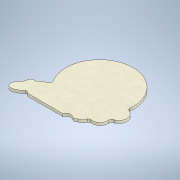
# Autodesk Inventor part: Mirage
Saved by Autodesk Inventor 2021 (Build 250183000, 183)
## iProperties
Created: 2023-03-16
Part Number: Mirage
Material: Paper
Document SubType Name: Modeling
Designer: Bradley
Density: 0.93 g/cm^3
Appearance: Cardboard - Chipboard
Author: Bradley
Autodesk Inventor part; units mm, degrees
ref_plane "YZ Plane" through (0, 0, 0) normal (1, 0, 0) x (0, 1, 0)
ref_plane "XZ Plane" through (0, 0, 0) normal (0, 1, 0) x (-1, 0, 0)
ref_plane "XY Plane" through (0, 0, 0) normal (0, 0, 1) x (1, 0, 0)
sketch "Sketch1" plane through (0, 0, 0) normal (0, 1, 0) x (-1, 0, 0)
  circle A0 centre (0, 0) radius 21.25
  spline S0 degree 4 poles (21.5183, 25.1806) (22.453, 25.9913) (23.7032, 27.2182) (26.5459, 28.7789) (29.6168, 28.3268) (30.3465, 26.3018) (30.4101, 25.2216) (29.2399, 22.7752) (28.2163, 21.9999) (26.3142, 19.6025) (27.1333, 18.9009) (26.1834, 17.1139) (25.1296, 16.6957) (23.2286, 17.0403) (23.092, 16.5163) (22.4952, 16.2276) (21.5363, 15.2647) (20.3375, 14.5722) (18.5927, 13.7313) (17.4687, 13.2094) (17.7562, 12.3127) (17.7525, 11.6795) knots 0 0 0 0 0 0.147812 0.205991 0.259658 0.311903 0.364532 0.419611 0.47324 0.524112 0.572905 0.618604 0.660693 0.697571 0.733333 0.769979 0.813271 0.85982 0.903638 1 1 1 1 1
  line L0 (19.4217, 26.1144) -> (-2.9724, 26.1144)
  arc A1 (-8.2059, 24.9208) -> (-2.9724, 26.1144) centre (-5.9805, 27.2337) ccw
  arc A2 (-8.2059, 24.9208) -> (-10.3084, 24.2647) centre (-9.036, 23.884) ccw
  arc A3 (-10.3084, 24.2647) -> (-13.559, 21.372) centre (-9.9206, 20.5562) ccw
  arc A4 (-14.9755, 20.5562) -> (-13.559, 21.372) centre (-15.0102, 22.2543) ccw
  arc A5 (-14.9755, 20.5562) -> (-20.9953, 15.492) centre (-16.0538, 15.728) ccw
  arc A6 (-22.7912, 13.2627) -> (-20.9953, 15.492) centre (-22.6152, 14.9589) ccw
  arc A7 (-22.7912, 13.2627) -> (-22.3249, 3.6593) centre (-20.712, 8.5507) ccw
  arc A8 (-21.1463, 2.097) -> (-22.3249, 3.6593) centre (-23.0249, 1.9055) ccw
  arc A9 (20.1143, 25.4202) -> (21.5183, 25.1806) centre (20.9688, 26.1937) ccw
  arc A10 (20.1143, 25.4202) -> (19.4217, 26.1144) centre (18.6329, 24.6347) ccw
  point P0 (22.9685, 26.4205)
  point P1 (25.0508, 27.7308)
  point P2 (27.6484, 28.4328)
  point P3 (29.4741, 27.848)
  point P4 (30.2229, 26.4204)
  point P5 (30.2226, 25.1799)
  point P6 (29.2861, 23.1437)
  point P7 (27.9754, 21.599)
  point P8 (26.7815, 19.633)
  point P9 (26.7813, 18.6968)
  point P10 (26.1258, 17.3627)
  point P11 (24.7452, 16.8477)
  point P12 (23.2946, 16.8009)
  point P13 (23.0144, 16.5675)
  point P14 (22.6406, 16.2638)
  point P15 (21.7049, 15.4917)
  point P16 (20.3013, 14.5798)
  point P17 (18.8504, 13.8542)
  point P18 (17.9846, 13.269)
  point P19 (17.7272, 12.637)
  dimension "d5" = 42.5
  constraints: 22 point on circle, 11 centre point, 2 end point, 2 horizontal, 1 coincident, 55 other
  measures "d5" diameter of A0
extrude "Extrusion1" add sketch "Sketch1" along normal mid plane 1.7
body "Solid1"
